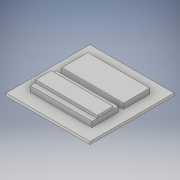
# Autodesk Inventor part: Assembly Station
Saved by Autodesk Inventor 2019.4 (Build 234330000, 330)
## iProperties
Created: 2020-11-10
Part Number: Assembly Station
Material: Generic
Document SubType Name: Modeling
Designer: caleb
Density: 1 g/cm^3
Appearance: Default
Author: caleb
Autodesk Inventor part; units mm, degrees
ref_plane "YZ Plane" through (0, 0, 0) normal (1, 0, 0) x (0, 1, 0)
ref_plane "XZ Plane" through (0, 0, 0) normal (0, 1, 0) x (-1, 0, 0)
ref_plane "XY Plane" through (0, 0, 0) normal (0, 0, 1) x (1, 0, 0)
sketch "Sketch1" plane through (0, 0, 0) normal (0, 1, 0) x (-1, 0, 0)
  line L0 (101.6, 101.6) -> (-101.6, 101.6)
  line L1 (-101.6, 101.6) -> (-101.6, -101.6)
  line L2 (-101.6, -101.6) -> (101.6, -101.6)
  line L3 (101.6, -101.6) -> (101.6, 101.6)
  point P0 (0, 0)
  dimension "d0" = 203.2
  dimension "d1" = 101.6
  dimension "d2" = 101.6
  constraints: 8 end point, 2 parallel, 2 perpendicular, 1 horizontal
  measures "d0" distance of L2.end L0.start
  measures "d1" distance from line of L0 point (0, 0)
  measures "d2" distance from line of L3 point (0, 0)
extrude "Extrusion1" add sketch "Sketch1" along normal blind 6.35
sketch "Sketch2" plane through (0, 6.35, 0) normal (0, 1, 0) x (1, 0, 0)
  line L0 (-74.6125, -69.85) -> (74.6125, -69.85)
  line L1 (74.6125, -69.85) -> (74.6125, -6.35)
  line L2 (74.6125, -6.35) -> (-74.6125, -6.35)
  line L3 (-74.6125, -6.35) -> (-74.6125, -69.85)
  line L4 (-101.6, -101.6) -> (101.6, -101.6) projected
  line L5 (101.6, -101.6) -> (101.6, 101.6) projected
  line L6 (-101.6, -101.6) -> (101.6, -101.6) projected
  line L7 (101.6, -101.6) -> (101.6, 101.6) projected
  line L8 (101.6, 101.6) -> (-101.6, 101.6) projected
  line L9 (-101.6, 101.6) -> (-101.6, -101.6) projected
  line L10 (-74.6125, 6.35) -> (74.6125, 6.35)
  line L11 (74.6125, 6.35) -> (74.6125, 69.85)
  line L12 (74.6125, 69.85) -> (-74.6125, 69.85)
  line L13 (-74.6125, 69.85) -> (-74.6125, 6.35)
  point P0 (0, 0)
  dimension "d5" = 149.225
  dimension "d6" = 63.5
  dimension "d7" = 26.9875
  dimension "d8" = 31.75
  dimension "d9" = 63.5
  dimension "d10" = 31.75
  constraints: 16 end point, 4 parallel, 2 horizontal, 2 perpendicular
  measures "d5" distance of L0.start L0.end
  measures "d6" distance of L2.end L0.start
  measures "d7" distance from line of L5 L0.end
  measures "d8" distance from line of L4 L0.end
  measures "d9" distance of L12.end L10.start
  measures "d10" distance from line of L8 L11.end
extrude "Extrusion2" add sketch "Sketch2" along normal blind 12.7 contours L3 L2 L1 L0 | L13 L12 L11 L10
sketch "Sketch3" plane through (0, 19.05, 0) normal (0, 1, 0) x (1, 0, 0)
  line L0 (-74.6125, -69.85) -> (-74.6125, -6.35) projected
  line L1 (74.7769, -57.15) -> (-74.6125, -57.15)
  line L2 (-74.6125, -57.15) -> (-74.6125, -19.05)
  line L3 (-74.6125, -19.05) -> (74.7769, -19.05)
  line L4 (74.7769, -19.05) -> (74.7769, -57.15)
  line L5 (74.6125, -69.85) -> (74.6125, -6.35) projected
  line L6 (-74.6125, -6.35) -> (-74.6125, -69.85) projected
  point P0 (0, 0)
  dimension "d13" = 38.1
  dimension "d14" = 12.7
  constraints: 8 end point, 2 parallel, 1 horizontal, 1 perpendicular, 1 point on line
  measures "d13" distance of L2.end L1.end
  measures "d14" distance of L0.start L1.end
extrude "Extrusion3" add sketch "Sketch3" along normal blind 6.35
body "Solid1"
